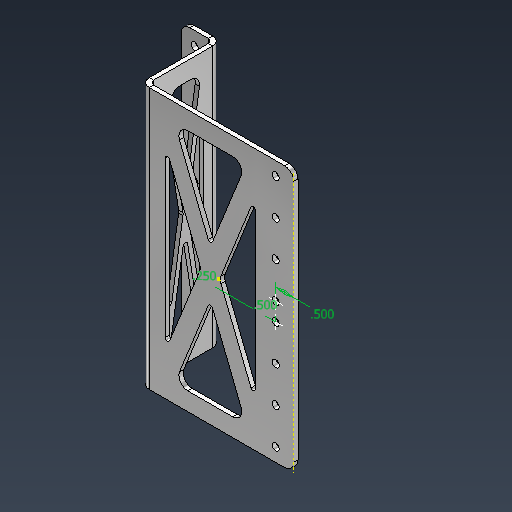
# Autodesk Inventor part: PLATE,MOUNT,BATTERY
Saved by Autodesk Inventor 2026 (Build 300175050, 175E)
## iProperties
Created: 2026-02-21
Part Number: PLATE,MOUNT,BATTERY
Material: Aluminum 3003-O
Document SubType Name: Sheet Metal
Designer: Jthib
Mass: 193.646 g
Surface Area: 537.262 cm^2
Volume: 70.7232 cm^3
Density: 2.73809 g/cm^3
Sheet Metal Rule: Default
Appearance: Aluminum - Polished
Author: Jthib
Autodesk Inventor part; units mm, degrees
ref_plane "YZ Plane" through (0, 0, 0) normal (1, 0, 0) x (0, 1, 0)
ref_plane "XZ Plane" through (0, 0, 0) normal (0, 1, 0) x (-1, 0, 0)
ref_plane "XY Plane" through (0, 0, 0) normal (0, 0, 1) x (1, 0, 0)
sketch "Sketch1" plane through (0, 0, 0) normal (0, 0, 1) x (1, 0, 0)
  line L0 (52.3875, -92.075) -> (-52.3875, -92.075)
  line L1 (-52.3875, -92.075) -> (-52.3875, 92.075)
  line L2 (-52.3875, 92.075) -> (52.3875, 92.075)
  line L3 (52.3875, 92.075) -> (52.3875, -92.075)
  line L4 (52.3875, -92.075) -> (-52.3875, 92.075) construction
  line L5 (-52.3875, -92.075) -> (52.3875, 92.075) construction
  point P0 (0, 0)
  dimension "d0" = 104.775
  dimension "d1" = 184.15
  measures "d0" distance of L1.end L2.end
  measures "d1" distance of L2.end L0.start
extrude "Plate1" add sketch "Sketch1" along normal blind 3.048
sketch "Sketch2" plane through (0, 0, 3.048) normal (0, 0, 1) x (1, 0, 0)
  line L0 (52.3875, 92.075) -> (52.3875, -92.075) construction
  point P0 (0, 0)
  point P1 (39.6875, -6.35)
  point P2 (39.6875, 6.35)
  dimension "d3" = 12.7
  dimension "d14" = 6.35
  dimension "d15" = 12.7
  constraints: 1 vertical alignment
  measures "d3" distance from line of L0 point (39.688, -6.35)
  measures "d14" vertical distance of point (0, 0) point (39.688, -6.35)
  measures "d15" distance of point (39.688, 6.35) point (39.688, -6.35)
hole "Hole1" at (39.6875, -6.35, 3.048) direction (0, 0, -1) diameter 5.1054 end through all start extended yes clearance for "Flat Head Machine Screw (82)" size "#10" standard "Ansi Unified Screw Threads"
hole "Hole2" at (39.6875, 6.35, 3.048) direction (0, 0, -1) diameter 5.1054 end through all start extended yes clearance for "Flat Head Machine Screw (82)" size "#10" standard "Ansi Unified Screw Threads"
pattern_linear "Rectangular Pattern2" count 4 spacing 25.4 along (0, -1, 0) of "Hole1"
pattern_linear "Rectangular Pattern3" count 4 spacing 25.4 along (0, 1, 0) of "Hole2"
sketch "Sketch3" plane through (-52.3875, 92.075, 0) normal (-1, 0, 0) x (0, -1, 0)
  line L0 (184.15, 0) -> (0, 0)
  line L1 (0, 0) -> (0, -47.752)
  line L2 (0, -47.752) -> (184.15, -47.752)
  line L3 (184.15, -47.752) -> (184.15, 0)
  constraints: 6 end point, 1 horizontal, 1 perpendicular, 1 vertical
edge flange "Flange1" height 50.8 angle 90 thickness 3.048 bend radius 3.048 thickness toward (-1, 0, 0) relief straight relief width 3.048 relief depth 1.524 edges at (-52.3875, 0, 0) wall of the first edge with corners at (-52.3875, -92.075, 0) (-52.3875, 92.075, 0) (-52.3875, 92.075, -47.752) (-52.3875, -92.075, -47.752)
bend "Bend1"
corner "Corner1"
sketch "Sketch4" plane through (-55.4355, -92.075, -47.752) normal (0, 0, -1) x (-1, 0, 0)
  line L0 (0, 184.15) -> (0, 0)
  line L1 (0, 0) -> (22.352, 0)
  line L2 (22.352, 0) -> (22.352, 184.15)
  line L3 (22.352, 184.15) -> (0, 184.15)
  constraints: 6 end point, 1 horizontal, 1 perpendicular, 1 vertical
edge flange "Flange2" height 25.4 angle 90 thickness 3.048 bend radius 3.048 thickness toward (0, 0, -1) relief straight relief width 3.048 relief depth 1.524 edges at (-55.4355, 0, -47.752) wall of the first edge with corners at (-55.4355, 92.075, -47.752) (-55.4355, -92.075, -47.752) (-77.7875, -92.075, -47.752) (-77.7875, 92.075, -47.752)
bend "Bend2"
corner "Corner2"
sketch "Sketch6" plane through (-77.7875, -92.075, -47.752) normal (0, 0, 1) x (1, 0, 0)
  line L0 (0, 184.15) -> (0, 0) construction
  line L1 (9.525, 174.625) -> (9.525, 9.525) construction
  point P0 (77.7875, 92.075)
  point P1 (9.525, 92.075)
  point P2 (0, 92.075)
  dimension "d59" = 9.525
  dimension "d60" = 165.1
  constraints: 2 coincident, 2 end point, 2 midpoint, 1 horizontal alignment, 1 vertical
  measures "d59" distance between parallel lines of L0 L1
  measures "d60" distance of L1.start L1.end
hole "Hole4" at (-68.2625, 82.55, -47.752) at (-68.2625, -82.55, -47.752) at (-68.2625, 0, -47.752) direction (0, 0, -1) diameter 5.1054 end through all start extended yes clearance for "Flat Head Machine Screw (82)" size "#10" standard "Ansi Unified Screw Threads"
sketch "Sketch7" plane through (-55.4355, -92.075, -3.048) normal (-1, 0, 0) x (0, 0, 1)
  line L0 (-35.052, 12.7) -> (-9.652, 12.7)
  line L1 (-9.652, 12.7) -> (-9.652, 171.45)
  line L2 (-9.652, 171.45) -> (-35.052, 171.45)
  line L3 (-35.052, 171.45) -> (-35.052, 12.7)
  line L4 (-35.052, 12.7) -> (-9.652, 171.45) construction
  line L5 (-9.652, 12.7) -> (-35.052, 171.45) construction
  line L6 (-58.5216, 92.075) -> (16.8656, 92.075) construction
  line L7 (3.048, 220.98) -> (3.048, -36.83) construction
  line L8 (-33.5086, 12.7) -> (-9.652, 161.8039)
  line L9 (-11.1954, 171.45) -> (-35.052, 22.3461)
  line L10 (-9.652, 22.3461) -> (-33.5086, 171.45)
  line L11 (-11.1954, 12.7) -> (-35.052, 161.8039)
  point P0 (3.048, 92.075)
  point P1 (-22.352, 92.075)
  point P2 (-22.352, 82.4289)
  point P3 (-23.8954, 92.075)
  point P4 (-20.8086, 92.075)
  point P5 (-22.352, 101.7211)
  dimension "d68" = 25.4
  dimension "d69" = 158.75
  dimension "d70" = 25.4
  dimension "d74" = 1.524
  dimension "d82" = 3.048
  constraints: 20 end point, 9 point on line, 3 parallel, 2 midpoint, 1 horizontal, 1 perpendicular, 2 other
  measures "d68" distance from line of L7 point (-22.352, 92.075)
  measures "d69" distance of L0.end L1.end
  measures "d70" distance of L1.end L2.end
  measures "d74" distance between parallel lines of L10 L5
  measures "d82" distance between parallel lines of L8 L9
extrude "Cut1" cut sketch "Sketch7" against normal blind 3.048 contours L8 L11 L0 | L3 L11 L9 | L8 L1 L10 | L10 L2 L9
sketch "Sketch8" plane through (0, 0, 3.048) normal (0, 0, 1) x (1, 0, 0)
  line L0 (-38.1, -79.375) -> (25.4, -79.375)
  line L1 (25.4, -79.375) -> (25.4, 79.375)
  line L2 (25.4, 79.375) -> (-38.1, 79.375)
  line L3 (-38.1, 79.375) -> (-38.1, -79.375)
  line L4 (-38.1, -79.375) -> (25.4, 79.375) construction
  line L5 (25.4, -79.375) -> (-38.1, 79.375) construction
  line L6 (-103.8225, 0) -> (78.4225, 0) construction
  line L7 (25.4, -62.961) -> (-31.5344, 79.375)
  line L8 (18.8344, -79.375) -> (-38.1, 62.961)
  line L9 (-38.1, -62.961) -> (18.8344, 79.375)
  line L10 (-31.5344, -79.375) -> (25.4, 62.961)
  point P0 (0, 0)
  point P1 (-6.35, 0)
  point P2 (-6.35, -16.414)
  point P3 (0.2156, 0)
  point P4 (-12.9156, 0)
  point P5 (-6.35, 16.414)
  dimension "d75" = 6.35
  dimension "d76" = 63.5
  dimension "d77" = 158.75
  dimension "d78" = 12.192
  dimension "d79" = 12.192
  constraints: 20 end point, 9 point on line, 6 parallel, 2 midpoint, 1 horizontal, 1 perpendicular, 2 other
  measures "d75" distance of point (0, 0) point (-6.35, 0)
  measures "d76" distance of L1.end L2.end
  measures "d77" distance of L0.end L1.end
  measures "d78" distance between parallel lines of L7 L8
  measures "d79" distance between parallel lines of L10 L9
extrude "Cut2" cut sketch "Sketch8" against normal blind 3.048 contours L10 L8 L0 | L3 L8 L9 | L10 L1 L7 | L7 L2 L9
fillet "Corner Round1" radius 6.35 4 edges at (52.3875, -92.075, 1.524) (52.3875, 92.075, 1.524) (-77.7875, 92.075, -49.276) (-77.7875, -92.075, -49.276)
fillet "Corner Round2" radius 6.35 12 edges at (-12.9156, 0, 1.524) (0.2156, 0, 1.524) (18.8344, 79.375, 1.524) (-31.5344, 79.375, 1.524) (18.8344, -79.375, 1.524) (-31.5344, -79.375, 1.524) (-53.9115, -79.375, -14.2434) (-53.9115, -79.375, -36.5566) (-53.9115, 79.375, -36.5566) (-53.9115, 79.375, -14.2434) (-53.9115, 0, -23.8566) (-53.9115, 0, -26.9434)
fillet "Corner Round2" radius 1.5875 12 edges at (-53.9115, 69.7289, -12.7) (-53.9115, -69.7289, -12.7) (-53.9115, -69.7289, -38.1) (-53.9115, -9.6461, -25.4) (-53.9115, 9.6461, -25.4) (-53.9115, 69.7289, -38.1) (-38.1, -62.961, 1.524) (-38.1, 62.961, 1.524) (25.4, -62.961, 1.524) (25.4, 62.961, 1.524) (-6.35, 16.414, 1.524) (-6.35, -16.414, 1.524)
equation "\"d9\" = Thickness"
equation "\"d68\" = 0.5 * d34"
equation "\"d70\" = d68"
equation "\"d74\" = d71"
equation "\"d82\" = 2 * d74"
equation "\"d72\" = Thickness"
equation "\"d78\" = 4 * Thickness"
equation "\"d79\" = d78"
equation "\"d80\" = Thickness"
equation "\"d2\" = Thickness"
equation "\"d30\" = BendReliefWidth"
equation "\"d31\" = BendReliefDepth"
equation "\"d32\" = MinimumRemnant"
equation "\"d33\" = TransitionRadius"
equation "\"d36\" = BendRadius"
equation "\"d37\" = CornerReliefSize"
equation "\"d38\" = GapSize"
equation "\"d39\" = JacobiRadiusSize"
equation "\"d40\" = BendReliefWidth"
equation "\"d41\" = BendReliefDepth"
equation "\"d42\" = MinimumRemnant"
equation "\"d43\" = TransitionRadius"
equation "\"d46\" = BendRadius"
equation "\"d47\" = CornerReliefSize"
equation "\"d48\" = GapSize"
equation "\"d49\" = JacobiRadiusSize"
equation "\"BendRadius\" = Thickness"
equation "\"BendReliefWidth\" = Thickness"
equation "\"BendReliefDepth\" = 0.5 * Thickness"
equation "\"CornerReliefSize\" = 4 * Thickness"
equation "\"MinimumRemnant\" = 2 * Thickness"
equation "\"TransitionRadius\" = BendRadius"
equation "\"JacobiRadiusSize\" = BendRadius"
equation "\"GapSize\" = Thickness"
equation "\"d71\" = 0.5 * Thickness"
equation "\"Thickness\" = 3.048"
equation "\"d34\" = 50.8"
body "Solid1"
